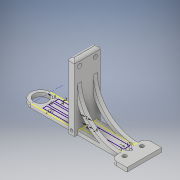
# Autodesk Inventor part: TapeMeasureBracketSideServo
Saved by Autodesk Inventor 2019 (Build 230136000, 136)
## iProperties
Created: 2018-11-04
Part Number: TapeMeasureBracketSideServo
Material: Generic
Document SubType Name: Modeling
Designer: mrhftc
Density: 1 g/cm^3
Appearance: Default
Author: mrhftc
Autodesk Inventor part; units mm, degrees
ref_plane "YZ Plane" through (0, 0, 0) normal (1, 0, 0) x (0, 1, 0)
ref_plane "XZ Plane" through (0, 0, 0) normal (0, 1, 0) x (-1, 0, 0)
ref_plane "XY Plane" through (0, 0, 0) normal (0, 0, 1) x (1, 0, 0)
sketch "Main Sketch" plane through (0, 0, 0) normal (0, 1, 0) x (-1, 0, 0)
  line L0 (-57.375, -12.0472) -> (-57.375, 12.0472)
  line L1 (-57.375, 12.0472) -> (47.625, -10) construction
  line L2 (47.625, 10) -> (-57.375, -12.0472) construction
  circle A0 centre (47.625, 0) radius 7
  arc A1 (47.625, -10) -> (47.625, 10) centre (47.625, 0) ccw
  line L3 (-40.875, 17.5) -> (-57.375, 17.5)
  line L4 (-57.375, 17.5) -> (-57.375, -17.5)
  line L5 (-57.375, -17.5) -> (-40.875, -17.5)
  line L6 (-40.875, 17.5) -> (-57.375, -17.5) construction
  line L7 (-57.375, 17.5) -> (-40.875, -17.5) construction
  line L8 (47.625, -10) -> (-40.875, -10)
  line L9 (-40.875, -17.5) -> (-40.875, -10)
  line L10 (-40.875, 10) -> (-40.875, 17.5)
  line L11 (-40.875, 10) -> (47.625, 10)
  point P0 (0, 0)
  point P1 (-49.125, 0)
  dimension "d3" = 14
  dimension "d4" = 105
  dimension "d13" = 16.5
  dimension "d14" = 35
  dimension "d15" = 0
  dimension "d18" = 20
  constraints: 24 end point, 4 parallel, 2 centre point, 2 horizontal, 2 midpoint, 2 point on circle, 2 point on line, 1 coincident, 1 perpendicular
  measures "d3" diameter of A0
  measures "d4" distance from line of L0 A0.centre
  measures "d13" distance of L4.end L5.end
  measures "d14" distance of L3.end L4.end
  measures "d15" distance between parallel lines of L0 L4
  measures "d18" distance between parallel lines of L11 L8
extrude "Main Extrusion" add sketch "Main Sketch" along normal blind 4
sketch "Screw Holes Sketch" plane through (0, 4, 0) normal (0, 1, 0) x (1, 0, 0)
  circle A0 centre (46.125, -8.75) radius 2
  line L0 (57.375, 17.5) -> (40.875, 17.5) projected
  line L1 (40.875, -17.5) -> (57.375, -17.5) projected
  line L2 (35.2664, 0) -> (65.7891, 0)
  line L3 (51.375, -27.0398) -> (51.375, 30.2346) construction
  line L4 (57.375, -17.5) -> (57.375, 17.5) projected
  line L5 (40.875, -10) -> (40.875, -17.5) projected
  circle A1 centre (46.125, 8.75) radius 2
  line L6 (51.375, 27.0398) -> (51.375, -30.2346) construction
  point P0 (0, 0)
  dimension "d21" = 4
  dimension "d22" = 35
  dimension "d23" = 6
  dimension "d24" = 5.25
  dimension "d25" = 5.25
  dimension "d26" = 10.5
  dimension "d27" = 8.75
  dimension "d28" = 17.5
  constraints: 6 end point, 3 symmetric about line, 2 centre point, 1 horizontal, 1 vertical, 1 other
  measures "d21" diameter of A0
  measures "d22" distance between parallel lines of L0 L1
  measures "d23" distance between parallel lines of L4 L3
  measures "d24" distance from line of L3 A0.centre
  measures "d25" distance from line of L5 A0.centre
  measures "d26" distance between parallel lines of L3 L5
  measures "d27" distance from line of L1 A0.centre
  measures "d28" diameter of A0.centre L2
extrude "Screw Holes Cut" cut sketch "Screw Holes Sketch" against normal through all
fillet "Smoooooooooooooooooth" radius 6 2 edges at (40.875, 2, -17.5) (40.875, 2, 17.5)
sketch "Side Axel Hole Sketch" plane through (-47.625, 0, 10) normal (0, 0, 1) x (1, 0, 0)
  line L0 (88.5, 4) -> (88.5, 0) projected
  line L1 (0, 0) -> (0, 4) projected
  line L2 (44.25, -12.0383) -> (44.25, 22.7681) construction
  line L3 (88.5, 0) -> (0, 0) projected
  line L4 (0, 4) -> (88.5, 4) projected
  circle A0 centre (44.25, 4) radius 1.5
  point P0 (47.625, 0)
  dimension "d32" = 88.5
  dimension "d33" = 44.25
  dimension "d34" = 44.25
  dimension "d35" = 4
  dimension "d41" = 3
  constraints: 2 end point, 1 centre point, 1 midpoint, 1 vertical
  measures "d32" distance between parallel lines of L0 L1
  measures "d33" distance between parallel lines of L1 L2
  measures "d34" distance between parallel lines of L0 L2
  measures "d35" distance between parallel lines of L3 L4
  measures "d41" diameter of A0
sketch "Sketch7" plane through (0, 4, 0) normal (0, 1, 0) x (1, 0, 0)
  line L0 (-47.625, -10) -> (40.875, -10) construction
  line L1 (-3.375, -10) -> (-3.375, 33.3565) construction
  line L2 (-0.3194, -13) -> (-6.4306, -13)
  line L3 (-6.4306, -13) -> (-6.4306, 13)
  line L4 (-6.4306, 13) -> (-0.3194, 13)
  line L5 (-0.3194, 13) -> (-0.3194, -13)
  line L6 (-0.3194, -13) -> (-6.4306, 13) construction
  line L7 (-6.4306, -13) -> (-0.3194, 13) construction
  point P0 (0, 0)
  point P1 (-3.375, 0)
  dimension "d47" = 26
  constraints: 14 end point, 3 midpoint, 2 parallel, 1 horizontal, 1 perpendicular, 1 point on line, 1 vertical
  measures "d47" distance between parallel lines of L2 L4
extrude "Servo Mount Extrusion" add sketch "Sketch7" along normal blind 62.8 and the other way blind 4
extrude "Side Axel Cut" cut sketch "Side Axel Hole Sketch" along normal through all both and the other way through all contours A0 L4 | L4 A0
sketch "Sketch8" plane through (-6.4306, 4, -10) normal (-1, 0, 0) x (0, 0, 1)
  line L0 (23, 62.8) -> (23, -4) construction
  line L1 (-3, 62.8) -> (23, 62.8) construction
  line L2 (-3, 62.8) -> (-3, -4) construction
  circle A0 centre (2, 55.8) radius 2
  circle A1 centre (18, 55.8) radius 2
  point P0 (10, -4)
  dimension "d54" = 4
  dimension "d55" = 4
  dimension "d56" = 16
  dimension "d57" = 7
  dimension "d58" = 7
  dimension "d59" = 5
  dimension "d60" = 5
  constraints: 2 centre point
  measures "d54" diameter of A0
  measures "d55" diameter of A1
  measures "d56" distance of A1.centre A0.centre
  measures "d57" distance from line of L1 A0.centre
  measures "d58" distance from line of L1 A1.centre
  measures "d59" distance from line of L0 A1.centre
  measures "d60" distance from line of L2 A0.centre
extrude "Mount Holes Cut" cut sketch "Sketch8" against normal through all
fillet "Support" radius 41 1 edges at (-0.3194, 4, 0)
fillet "lil hat" radius 3 4 edges at (-0.3194, 66.8, 0) (-3.375, 66.8, -13) (-6.4306, 66.8, 0) (-3.375, 66.8, 13)
ref_plane "Lifted XZ Plane" through (0, 45, 0) normal (0, -1, 0) x (1, 0, 0)
sketch "Support Center Sketch" plane through (0, 45, 0) normal (0, -1, 0) x (1, 0, 0)
  line L0 (40.6806, 10) -> (40.6806, -10) projected
  line L1 (-0.3194, -6) -> (40.6806, -6)
  line L2 (40.6806, -6) -> (40.6806, 6)
  line L3 (40.6806, 6) -> (-0.3194, 6)
  line L4 (-0.3194, 6) -> (-0.3194, -6)
  line L5 (-0.3194, -10) -> (40.6806, -10) projected
  line L6 (40.6806, 10) -> (-0.3194, 10) projected
  point P0 (0, 0)
  dimension "d66" = 41
  dimension "d67" = 4
  dimension "d68" = 4
  dimension "d69" = 12
  constraints: 8 end point, 2 parallel, 1 horizontal, 1 perpendicular, 1 point on line
  measures "d66" distance between parallel lines of L0 L4
  measures "d67" distance between parallel lines of L1 L5
  measures "d68" distance between parallel lines of L6 L3
  measures "d69" distance between parallel lines of L3 L1
extrude "Support Center Cut" cut sketch "Support Center Sketch" along normal blind 41
sketch "Support Side Cut Sketch" plane through (40.875, 0, -10) normal (0, 0, -1) x (-1, 0, 0)
  arc A0 (0.1944, 4) -> (41.1944, 45) centre (0.1944, 45) ccw construction
  arc A1 (0.1944, 4) -> (41.1944, 45) centre (0.1944, 45) ccw projected
  arc A2 (18.7416, 4) -> (41.1944, 26.4528) centre (0.1944, 45) ccw
  line L0 (-6, 4) -> (0, 4) projected
  line L1 (41.1944, 0) -> (41.1944, 45) projected
  line L2 (41.1944, 0) -> (0, 0) projected
  line L3 (41.1944, 26.4528) -> (41.1944, 4)
  line L4 (0, 4) -> (0.1944, 4)
  line L5 (18.7416, 4) -> (41.1944, 4)
  point P0 (40.875, 0)
  dimension "d72" = 41
  dimension "d73" = 45
  dimension "d75" = 4
  constraints: 6 end point, 5 point on circle, 2 centre point, 2 horizontal, 2 point on line, 1 coincident, 1 collinear, 1 concentric
  measures "d72" distance of A0.centre L1.end
  measures "d73" radius of A2
  measures "d75" distance between parallel lines of L2 L5
extrude "Support Side Cut" cut sketch "Support Side Cut Sketch" against normal through all
sketch "Sketch11" plane through (0, 4, 0) normal (0, 1, 0) x (1, 0, 0)
  line L0 (-37.625, 4) -> (-8.4306, 4)
  line L1 (-8.4306, 4) -> (-8.4306, 8)
  line L2 (-8.4306, 8) -> (-37.625, 8)
  line L3 (-37.625, 8) -> (-37.625, 4)
  line L4 (-6.4306, 10) -> (-47.625, 10) projected
  line L5 (-6.4306, -10) -> (-6.4306, 10) projected
  line L6 (-47.625, -13.767) -> (-47.625, 22.327) construction
  line L7 (-37.625, -2) -> (-8.4306, -2)
  line L8 (-8.4306, -2) -> (-8.4306, 2)
  line L9 (-8.4306, 2) -> (-37.625, 2)
  line L10 (-37.625, 2) -> (-37.625, -2)
  line L11 (-37.625, -8) -> (-8.4306, -8)
  line L12 (-8.4306, -8) -> (-8.4306, -4)
  line L13 (-8.4306, -4) -> (-37.625, -4)
  line L14 (-37.625, -4) -> (-37.625, -8)
  line L15 (-47.625, -10) -> (-6.4306, -10) projected
  line L16 (39.4306, 3) -> (1.6806, 3)
  line L17 (1.6806, 3) -> (1.6806, -3)
  line L18 (1.6806, -3) -> (39.4306, -3)
  line L19 (39.4306, -3) -> (39.4306, 3)
  line L20 (40.6806, -6) -> (-0.3194, -6) projected
  line L21 (-0.3194, 6) -> (40.6806, 6) projected
  line L22 (-0.3194, 10) -> (-0.3194, -10) projected
  line L23 (40.6806, 6) -> (40.6806, 10) projected
  point P0 (0, 0)
  dimension "d78" = 2
  dimension "d79" = 2
  dimension "d80" = 10
  dimension "d81" = 4
  dimension "d84" = 6
  dimension "d89" = 2
  dimension "d90" = 6
  dimension "d91" = 3
  dimension "d92" = 3
  dimension "d93" = 2
  dimension "d94" = 1.25
  constraints: 34 end point, 4 parallel, 3 vertical, 2 horizontal, 2 perpendicular, 16 other
  measures "d78" distance between parallel lines of L4 L2
  measures "d79" distance between parallel lines of L5 L1
  measures "d80" distance between parallel lines of L3 L6
  measures "d81" distance between parallel lines of L0 L2
  measures "d84" distance of L0.start L7.start
  measures "d89" distance between parallel lines of L15 L11
  measures "d90" distance between parallel lines of L16 L18
  measures "d91" distance between parallel lines of L18 L20
  measures "d92" distance between parallel lines of L21 L16
  measures "d93" distance between parallel lines of L17 L22
  measures "d94" distance between parallel lines of L23 L19
body "Solid3"
